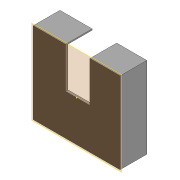
# Autodesk Inventor part: Part2
Saved by Autodesk Inventor 2018.1 (Build 221171000, 171)
## iProperties
Created: 2018-02-22
Part Number: Part2
Material: Generic
Document SubType Name: Modeling
Designer: RoboJackets
Density: 1 g/cm^3
Appearance: Default
Author: RoboJackets
Autodesk Inventor part; units mm, degrees
ref_plane "YZ Plane" through (0, 0, 0) normal (1, 0, 0) x (0, 1, 0)
ref_plane "XZ Plane" through (0, 0, 0) normal (0, 1, 0) x (-1, 0, 0)
ref_plane "XY Plane" through (0, 0, 0) normal (0, 0, 1) x (1, 0, 0)
ref_plane "Work Plane1" through (0, 0, 0) normal (0, 0, 1) x (1, 0, 0)
sketch "Sketch1" plane through (0, 0, 0) normal (0, 0, 1) x (1, 0, 0)
  line L0 (-44.1325, -41.275) -> (44.1325, -41.275)
  line L1 (44.1325, -41.275) -> (44.1325, 41.275)
  line L2 (44.1325, 41.275) -> (-44.1325, 41.275)
  line L3 (-44.1325, 41.275) -> (-44.1325, -41.275)
  line L4 (-44.1325, -41.275) -> (44.1325, 41.275) construction
  line L5 (44.1325, -41.275) -> (-44.1325, 41.275) construction
  line L6 (-45.4025, -42.545) -> (45.4025, -42.545)
  line L7 (45.4025, -42.545) -> (45.4025, 42.545)
  line L8 (45.4025, 42.545) -> (-45.4025, 42.545)
  line L9 (-45.4025, 42.545) -> (-45.4025, -42.545)
  line L10 (-45.4025, -42.545) -> (45.4025, 42.545) construction
  line L11 (45.4025, -42.545) -> (-45.4025, 42.545) construction
  point P0 (0, 0)
  dimension "d1" = 88.265
  dimension "d2" = 82.55
  dimension "d3" = 90.805
  dimension "d4" = 85.09
  constraints: 24 end point, 4 midpoint, 4 parallel, 2 horizontal, 2 perpendicular
  measures "d1" distance of L2.end L1.end
  measures "d2" distance between parallel lines of L0 L2
  measures "d3" distance of L8.end L7.end
  measures "d4" distance between parallel lines of L6 L8
extrude "Extrusion1" add sketch "Sketch1" against normal blind 27.94
sketch "Sketch2" plane through (0, 0, 0) normal (0, 0, 1) x (1, 0, 0)
  line L0 (44.1325, 41.275) -> (-44.1325, 41.275) projected
  line L1 (-44.1325, -41.275) -> (44.1325, -41.275) projected
  line L2 (-44.1325, 41.275) -> (44.1325, 41.275)
  line L3 (44.1325, 41.275) -> (44.1325, -41.275)
  line L4 (44.1325, -41.275) -> (-44.1325, -41.275)
  line L5 (-44.1325, -41.275) -> (-44.1325, 41.275)
  point P0 (0, 0)
  constraints: 8 end point, 2 parallel, 1 horizontal, 1 perpendicular
extrude "Extrusion2" add sketch "Sketch2" against normal blind 2.54
sketch "Sketch5" plane through (0, 0, 0) normal (0, 0, 1) x (1, 0, 0)
  line L0 (-45.4025, 42.545) -> (45.4025, 42.545) projected
  line L1 (-5.1231, 42.545) -> (4.8162, 42.545)
  line L2 (4.8162, 42.545) -> (4.8162, 17.0095)
  line L3 (4.8162, 17.0095) -> (-5.1231, 17.0095)
  line L4 (-5.1231, 17.0095) -> (-5.1231, 42.545)
  point P0 (0, 0)
  constraints: 8 end point, 2 parallel, 1 horizontal, 1 perpendicular, 1 point on line
extrude "Extrusion3" cut sketch "Sketch5" against normal up to next
sketch "Sketch6" plane through (0, 0, 0) normal (0, 0, 1) x (1, 0, 0)
  line L0 (-45.4025, 42.545) -> (-5.1231, 42.545) projected
  line L1 (-11.7648, 42.545) -> (10.5336, 42.545)
  line L2 (10.5336, 42.545) -> (10.5336, 5.472)
  line L3 (10.5336, 5.472) -> (-11.7648, 5.472)
  line L4 (-11.7648, 5.472) -> (-11.7648, 42.545)
  point P0 (0, 0)
  constraints: 8 end point, 2 parallel, 1 horizontal, 1 perpendicular, 1 point on line
extrude "Extrusion4" cut sketch "Sketch6" against normal up to next
sketch "Sketch7" plane through (0, 0, 0) normal (0, 0, 1) x (1, 0, 0)
  line L0 (13.9536, 42.6816) -> (-11.7648, 42.6816)
  line L1 (-11.7648, 42.6816) -> (-11.7648, 0)
  line L2 (-11.7648, 0) -> (13.9536, 0)
  line L3 (13.9536, 0) -> (13.9536, 42.6816)
  point P0 (0, 0)
  constraints: 8 end point, 2 parallel, 1 horizontal, 1 perpendicular
extrude "Extrusion5" cut sketch "Sketch7" against normal up to next
sketch "Sketch8" plane through (0, 0, 0) normal (0, 0, 1) x (1, 0, 0)
  point P0 (0, 0)
body "Solid1"
